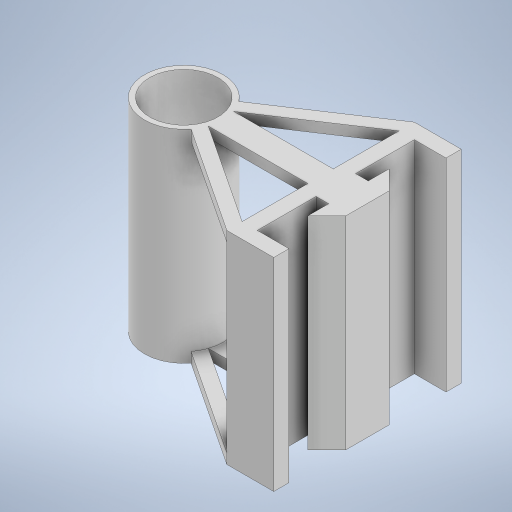
# Autodesk Inventor part: laser-solo
Saved by Autodesk Inventor 2023 (Build 270158000, 158)
## iProperties
Created: 2023-03-15
Part Number: laser-solo
Material: Ogólny
Document SubType Name: Modeling
Designer: kamil
Density: 1 g/cm^3
Appearance: Domyślna
Author: kamil
Autodesk Inventor part; units mm, degrees
ref_plane "YZ Plane" through (0, 0, 0) normal (1, 0, 0) x (0, 1, 0)
ref_plane "XZ Plane" through (0, 0, 0) normal (0, 1, 0) x (-1, 0, 0)
ref_plane "XY Plane" through (0, 0, 0) normal (0, 0, 1) x (1, 0, 0)
sketch "Szkic1" plane through (0, 0, 0) normal (0, 1, 0) x (-1, 0, 0)
  line L0 (3, 18.5) -> (-6.25, 18.5)
  line L1 (-6.25, 18.5) -> (-6.25, 15.5)
  line L2 (-6.25, 15.5) -> (0, 15.5)
  line L3 (0, 15.5) -> (0, -15.5)
  line L4 (0, -15.5) -> (-6.25, -15.5)
  line L5 (-6.25, -15.5) -> (-6.25, -18.5)
  line L6 (-6.25, -18.5) -> (3, -18.5)
  line L7 (3, -18.5) -> (3, 18.5)
  line L8 (3, 0) -> (0, 0) construction
  line L9 (0, 3.9) -> (-2.5, 3.9)
  line L10 (-2.5, 3.9) -> (-2.5, 8)
  line L11 (-2.5, 8) -> (-2.5, 8)
  line L12 (-2.5, 8) -> (-6.25, 4.25)
  line L13 (-6.25, 4.25) -> (-6.25, -4.25)
  line L14 (-6.25, -4.25) -> (-2.5, -8)
  line L15 (-2.5, -8) -> (-2.5, -8)
  line L16 (-2.5, -8) -> (-2.5, -3.9)
  line L17 (-2.5, -3.9) -> (0, -3.9)
  line L18 (-2.5, 3.9) -> (-2.5, -3.9) construction
  line L19 (-2.5, 0) -> (-6.25, 0) construction
  line L20 (3, 18.5) -> (3, 15.5)
  line L21 (3, -15.5) -> (3, -18.5)
  line L22 (3, -18.5) -> (3, 18.5)
  circle A0 centre (30, 0) radius 7.75
  circle A1 centre (30, 0) radius 6.75
  line L23 (3, 18.5) -> (23.8501, 4.7161)
  line L24 (22.6643, 2.5) -> (3, 15.5)
  line L25 (3, -15.5) -> (22.6643, -2.5)
  line L26 (3, -18.5) -> (23.8501, -4.7161)
  line L27 (22.6643, 2.5) -> (3, 2.5)
  line L28 (22.6643, -2.5) -> (3, -2.5)
  point P0 (0, 0)
  point P1 (1.5, -15)
  point P2 (1.5, 18)
  point P3 (1.5, 0)
  point P4 (3, 2.5)
  dimension "d1" = 7.8
  dimension "d3" = 16
  dimension "d4" = 2.5
  dimension "d6" = 3
  dimension "d7" = 3
  dimension "d11" = 8.5
  dimension "d12" = 6.25
  dimension "d26" = 31
  dimension "d42" = 13.5
  dimension "d43" = 15.5
  dimension "d44" = 30
  dimension "d45" = 5
  constraints: 58 end point, 13 perpendicular, 7 point on line, 6 parallel, 5 midpoint, 4 point on circle, 3 horizontal alignment, 3 vertical alignment, 2 centre point, 2 horizontal, 1 coincident, 1 vertical, 8 other
  measures "d1" distance between parallel lines of L17 L9
  measures "d3" distance between parallel lines of L11 L15
  measures "d4" distance between parallel lines of L3 L16
  measures "d6" distance of L0.end L1.end
  measures "d7" distance between parallel lines of L7 L3
  measures "d11" distance of L12.end L13.end
  measures "d12" distance between parallel lines of L13 L3
  measures "d26" distance between parallel lines of L2 L4
  measures "d42" diameter of A1
  measures "d43" diameter of A0
  measures "d44" distance of L8.end A0.centre
  measures "d45" distance between parallel lines of L28 L27
extrude "Wyciągnięcie proste2" add sketch "Szkic1" along normal blind 40 contours L7 L6 L5 L4 L3 L2 L1 L0 | L23 A0 L24 L7 | A0 | L27 A0 L28 L7 | A0 L26 L7 L25 | L3 L17 L16 L14 L13 L12 L10 L9
extrude "Wyciągnięcie proste7" cut sketch "Szkic1" along normal blind 38 contours L23 A0 L24 L7 | L27 A0 L28 L7 | A0 L26 L7 L25
extrude "Wyciągnięcie proste8" add sketch "Szkic1" along normal blind 2 contours L23 A0 L24 L7 | L27 A0 L28 L7 | A0 L26 L7 L25
